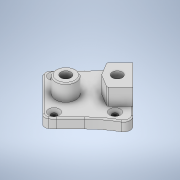
# Autodesk Inventor part: LegPin_Middle_v1
Saved by Autodesk Inventor 2020.3 (Build 243373000, 373)
## iProperties
Created: 2021-03-02
Part Number: LegPin_Middle_v1
Material: Generic
Document SubType Name: Modeling
Designer: sanyi
Density: 1 g/cm^3
Appearance: Default
Author: sanyi
Autodesk Inventor part; units mm, degrees
ref_plane "YZ Plane" through (0, 0, 0) normal (1, 0, 0) x (0, 1, 0)
ref_plane "XZ Plane" through (0, 0, 0) normal (0, 1, 0) x (-1, 0, 0)
ref_plane "XY Plane" through (0, 0, 0) normal (0, 0, 1) x (1, 0, 0)
sketch "Sketch1" plane through (0, 0, 0) normal (0, 1, 0) x (-1, 0, 0)
  line L0 (0, 114.5515) -> (0, -115.3375) construction
  line L1 (119.911, 0) -> (-136.2846, 0) construction
  line L2 (65, 45) -> (30.4932, 45) construction
  line L3 (-65, 45) -> (-65, 10.4932) construction
  line L4 (-65, -45) -> (-19.7, -45) construction
  line L5 (65, -45) -> (65, -10.4932) construction
  line L6 (64.2599, -35.4918) -> (81.6548, -52.8866) construction
  line L7 (81.6548, -52.8866) -> (72.8866, -61.6548) construction
  line L8 (72.8866, -61.6548) -> (55.4918, -44.2599) construction
  line L9 (55.4918, -44.2599) -> (64.2599, -35.4918) construction
  line L10 (64.2599, 35.4918) -> (81.6548, 52.8866)
  line L11 (81.6548, 52.8866) -> (72.8866, 61.6548)
  line L12 (72.8866, 61.6548) -> (55.4918, 44.2599)
  line L13 (55.4918, 44.2599) -> (59.8759, 39.8759)
  line L14 (-55.4918, 44.2599) -> (-72.8866, 61.6548) construction
  line L15 (-72.8866, 61.6548) -> (-81.6548, 52.8866) construction
  line L16 (-81.6548, 52.8866) -> (-64.2599, 35.4918) construction
  line L17 (-64.2599, 35.4918) -> (-55.4918, 44.2599) construction
  line L18 (-55.4918, -44.2599) -> (-72.8866, -61.6548) construction
  line L19 (-72.8866, -61.6548) -> (-81.6548, -52.8866) construction
  line L20 (-81.6548, -52.8866) -> (-64.2599, -35.4918) construction
  line L21 (-64.2599, -35.4918) -> (-55.4918, -44.2599) construction
  line L22 (55, 30) -> (-15, 30) construction
  line L23 (-15, 30) -> (-15, -30) construction
  line L24 (-15, -30) -> (55, -30) construction
  line L25 (55, -30) -> (55, 30) construction
  line L26 (72.9574, 44.1892) -> (64.1892, 52.9574) construction
  line L27 (68.0783, 56.8464) -> (76.8464, 48.0783) construction
  circle A0 centre (72.4624, 52.4624) radius 4.25
  line L28 (72.9574, -44.1892) -> (64.1892, -52.9574) construction
  line L29 (76.8464, -48.0783) -> (68.0783, -56.8464) construction
  circle A1 centre (72.4624, -52.4624) radius 4.25 construction
  line L30 (-64.1892, 52.9574) -> (-72.9574, 44.1892) construction
  line L31 (-68.0783, 56.8464) -> (-76.8464, 48.0783) construction
  circle A2 centre (-72.4624, 52.4624) radius 4.25 construction
  line L32 (-72.9574, -44.1892) -> (-64.1892, -52.9574) construction
  line L33 (-76.8464, -48.0783) -> (-68.0783, -56.8464) construction
  circle A3 centre (-72.4624, -52.4624) radius 4.25 construction
  line L34 (6.8, 51.2) -> (-17.8, 51.2) construction
  line L35 (-17.8, 51.2) -> (-17.8, 38.8) construction
  line L36 (-17.8, 38.8) -> (6.8, 38.8) construction
  line L37 (6.8, 38.8) -> (6.8, 51.2) construction
  line L38 (6.8, -38.8) -> (-17.8, -38.8) construction
  line L39 (-17.8, -38.8) -> (-17.8, -51.2) construction
  line L40 (-17.8, -51.2) -> (6.8, -51.2) construction
  line L41 (6.8, -51.2) -> (6.8, -38.8) construction
  line L42 (6.8, 45) -> (-17.8, 45) construction
  line L43 (-5.5, 51.2) -> (-5.5, 38.8) construction
  line L44 (0, 51.2) -> (0, 38.8) construction
  line L45 (6.8, -45) -> (-17.8, -45) construction
  line L46 (-5.5, -38.8) -> (-5.5, -51.2) construction
  line L47 (0, -38.8) -> (0, -51.2) construction
  circle A4 centre (0, 45) radius 4.25 construction
  circle A5 centre (0, -45) radius 4.25 construction
  line L48 (20, 30) -> (20, -30) construction
  line L49 (8.8, 57.2) -> (-19.8, 57.2) construction
  line L50 (8.8, -57.2) -> (-19.8, -57.2) construction
  line L51 (8.8, 57.2) -> (8.8, 45) construction
  line L52 (-19.8, 57.2) -> (-19.8, 45) construction
  line L53 (8.8, -57.2) -> (8.8, -45) construction
  line L54 (-19.8, -57.2) -> (-19.8, -45) construction
  line L55 (65.8156, 63.069) -> (59.9466, 57.2)
  line L56 (83.069, 45.8156) -> (77.2, 39.9466)
  line L57 (64.1892, 52.9574) -> (59.9466, 57.2) construction
  line L58 (72.9574, 44.1892) -> (77.2, 39.9466) construction
  arc A6 (83.069, 45.8156) -> (65.8156, 63.069) centre (74.4423, 54.4423) ccw
  line L59 (-59.9466, 57.2) -> (-65.8156, 63.069) construction
  line L60 (-83.069, 45.8156) -> (-77.2, 39.9466) construction
  line L61 (-59.9466, 57.2) -> (-64.1892, 52.9574) construction
  line L62 (-77.2, 39.9466) -> (-72.9574, 44.1892) construction
  arc A7 (-65.8156, 63.069) -> (-83.069, 45.8156) centre (-74.4423, 54.4423) ccw construction
  line L63 (72.9574, -44.1892) -> (77.2, -39.9466) construction
  line L64 (77.2, -39.9466) -> (83.069, -45.8156) construction
  line L65 (64.1892, -52.9574) -> (59.9466, -57.2) construction
  line L66 (59.9466, -57.2) -> (65.8156, -63.069) construction
  arc A8 (65.8156, -63.069) -> (83.069, -45.8156) centre (74.4423, -54.4423) ccw construction
  line L67 (-72.9574, -44.1892) -> (-77.2, -39.9466) construction
  line L68 (-64.1892, -52.9574) -> (-59.9466, -57.2) construction
  line L69 (-59.9466, -57.2) -> (-65.8156, -63.069) construction
  line L70 (-77.2, -39.9466) -> (-83.069, -45.8156) construction
  arc A9 (-83.069, -45.8156) -> (-65.8156, -63.069) centre (-74.4423, -54.4423) ccw construction
  arc A10 (23.5363, -45) -> (8.8, -57.2) centre (23.5363, -60) ccw construction
  arc A11 (59.9466, -57.2) -> (30.4932, -45) centre (30.4932, -86.6534) ccw construction
  arc A12 (65, -10.4932) -> (77.2, -39.9466) centre (106.6534, -10.4932) ccw construction
  arc A13 (77.2, 39.9466) -> (65, 10.4932) centre (106.6534, 10.4932) ccw
  arc A14 (30.4932, 45) -> (59.9466, 57.2) centre (30.4932, 86.6534) ccw
  arc A15 (8.8, 57.2) -> (23.5363, 45) centre (23.5363, 60) ccw construction
  arc A16 (-65, 10.4932) -> (-77.2, 39.9466) centre (-106.6534, 10.4932) ccw construction
  arc A17 (-77.2, -39.9466) -> (-65, -10.4932) centre (-106.6534, -10.4932) ccw construction
  line L71 (72.4624, -52.4624) -> (-72.4624, -52.4624) construction
  line L72 (-72.4624, 52.4624) -> (72.4624, 52.4624) construction
  line L73 (-59.9466, 57.2) -> (-59.9466, 45) construction
  line L74 (-59.9466, -57.2) -> (-59.9466, -45) construction
  arc A18 (-19.8, -57.2) -> (-34.5363, -45) centre (-34.5363, -60) ccw construction
  arc A19 (-30.4932, -45) -> (-59.9466, -57.2) centre (-30.4932, -86.6534) ccw construction
  arc A20 (-34.5363, 45) -> (-33.0208, 45.0768) centre (-34.5363, 60) ccw construction
  arc A21 (-59.9466, 57.2) -> (-33.0208, 45.0768) centre (-30.4932, 86.6534) ccw construction
  line L75 (72.8866, 61.6548) -> (75.7151, 64.4832) construction
  line L76 (75.7151, 64.4832) -> (84.4832, 55.7151) construction
  line L77 (84.4832, 55.7151) -> (81.6548, 52.8866) construction
  line L78 (78.6142, 58.6142) -> (58.5324, 38.5324) construction
  line L79 (58.5324, -38.5324) -> (78.6142, -58.6142) construction
  line L80 (-78.6142, 58.6142) -> (-58.5324, 38.5324) construction
  line L81 (-78.6142, -58.6142) -> (-58.5324, -38.5324) construction
  line L82 (74.4423, 54.4423) -> (77.2707, 57.2707) construction
  line L83 (74.4423, -54.4423) -> (77.2707, -57.2707) construction
  line L84 (-74.4423, -54.4423) -> (-77.2707, -57.2707) construction
  line L85 (-74.4423, 54.4423) -> (-77.2707, 57.2707) construction
  line L86 (-19.7, 45) -> (-65, 45) construction
  line L87 (8.7, 45) -> (-19.7, 45) construction
  line L88 (8.7, -45) -> (23.5363, -45) construction
  line L89 (-19.7, -45) -> (8.7, -45) construction
  line L90 (81.6548, 52.8866) -> (85.4206, 49.1209)
  line L91 (72.8866, 61.6548) -> (69.1209, 65.4206)
  line L92 (79.4627, 55.0787) -> (74.6544, 50.2704) construction
  line L93 (70.2704, -54.6544) -> (75.0787, -59.4627) construction
  line L94 (0, -48.1) -> (6.8, -48.1) construction
  line L95 (-74.6544, -50.2704) -> (-79.4627, -55.0787) construction
  line L96 (-75.0787, 59.4627) -> (-70.2704, 54.6544) construction
  line L97 (0, 48.1) -> (6.8, 48.1) construction
  line L98 (81.6548, -52.8866) -> (85.4206, -49.1209) construction
  line L99 (72.8866, -61.6548) -> (69.1209, -65.4206) construction
  line L100 (-72.8866, -61.6548) -> (-69.1209, -65.4206) construction
  line L101 (-81.6548, -52.8866) -> (-85.4206, -49.1209) construction
  line L102 (-72.8866, 61.6548) -> (-69.1209, 65.4206) construction
  line L103 (-81.6548, 52.8866) -> (-85.4206, 49.1209) construction
  line L104 (30.4932, 45) -> (23.5363, 45) construction
  line L105 (23.5363, 45) -> (8.7, 45) construction
  arc A22 (-33.0208, 45.0768) -> (-30.4932, 45) centre (-30.4932, 86.6534) ccw construction
  arc A23 (-33.0208, 45.0768) -> (-19.8, 57.2) centre (-34.5363, 60) ccw construction
  line L106 (-21.6459, 42) -> (-51.6459, 42) construction
  line L107 (-51.6459, 42) -> (-51.6459, -42) construction
  line L108 (-51.6459, -42) -> (-21.6459, -42) construction
  line L109 (-21.6459, -42) -> (-21.6459, 42) construction
  line L110 (52, 27) -> (55, 27) construction
  line L111 (52, -27) -> (55, -27) construction
  line L112 (52, 27) -> (52, 30) construction
  line L113 (-12, 27) -> (-12, 30) construction
  line L114 (-12, 27) -> (-15, 27) construction
  line L115 (-15, -27) -> (-12, -27) construction
  line L116 (-12, -27) -> (-12, -30) construction
  line L117 (52, -27) -> (52, -30) construction
  line L118 (-19.1459, 10) -> (-20.6459, 10) construction
  line L119 (-20.6459, 10) -> (-20.6459, -10) construction
  line L120 (-20.6459, -10) -> (-19.1459, -10) construction
  line L121 (-19.1459, -10) -> (-19.1459, 10) construction
  line L122 (-19.1459, 0) -> (-20.6459, 0) construction
  line L123 (-36.6459, 42) -> (-36.6459, -42) construction
  line L124 (-52.6459, 10) -> (-54.1459, 10) construction
  line L125 (-54.1459, 10) -> (-54.1459, -10) construction
  line L126 (-54.1459, -10) -> (-52.6459, -10) construction
  line L127 (-52.6459, -10) -> (-52.6459, 10) construction
  line L128 (-52.6459, 0) -> (-54.1459, 0) construction
  line L129 (30.4932, -45) -> (65, -45) construction
  line L130 (23.5363, -45) -> (30.4932, -45) construction
  line L131 (65, -10.4932) -> (65, 10.4932) construction
  line L132 (65, 10.4932) -> (65, 45) construction
  arc A24 (68.1707, 26.4333) -> (64.2599, 35.4918) centre (54.8044, 26.0363) ccw
  arc A25 (55.4918, 44.2599) -> (46.4333, 48.1707) centre (46.0363, 34.8044) ccw
  arc A26 (64.2599, -35.4918) -> (68.1707, -26.4333) centre (54.8044, -26.0363) ccw construction
  arc A27 (46.4333, -48.1707) -> (55.4918, -44.2599) centre (46.0363, -34.8044) ccw construction
  arc A28 (-55.4918, -44.2599) -> (-46.4333, -48.1707) centre (-46.0363, -34.8044) ccw construction
  arc A29 (-68.1707, -26.4333) -> (-64.2599, -35.4918) centre (-54.8044, -26.0363) ccw construction
  arc A30 (-47.594, 48.6723) -> (-55.4918, 44.2599) centre (-43.7511, 32.5192) ccw construction
  arc A31 (-64.2599, 35.4918) -> (-68.1707, 26.4333) centre (-54.8044, 26.0363) ccw construction
  line L133 (-65, 10.4932) -> (-65, -10.4932) construction
  line L134 (-65, -10.4932) -> (-65, -45) construction
  line L135 (-55.4918, 44.2599) -> (-55.4918, -44.2599) construction
  arc A32 (-19.9504, 56.5) -> (-17.8, 51.2) centre (-15.1706, 55.3531) ccw construction
  arc A33 (6.8, 51.2) -> (8.9504, 56.5) centre (4.1706, 55.3531) ccw construction
  arc A34 (8.9504, -56.5) -> (6.8, -51.2) centre (4.1706, -55.3531) ccw construction
  arc A35 (-17.8, -51.2) -> (-19.9504, -56.5) centre (-15.1706, -55.3531) ccw construction
  line L136 (-17.8, 38.8) -> (-17.8, 32.8) construction
  line L137 (-17.8, 32.8) -> (6.8, 32.8) construction
  line L138 (6.8, 32.8) -> (6.8, 38.8) construction
  line L139 (-17.8, -38.8) -> (-17.8, -32.8) construction
  line L140 (-17.8, -32.8) -> (6.8, -32.8) construction
  line L141 (6.8, -32.8) -> (6.8, -38.8) construction
  line L142 (81.4426, 48.4319) -> (68.4319, 61.4426) construction
  line L143 (68.4319, 61.4426) -> (55.704, 48.7147) construction
  line L144 (55.704, 48.7147) -> (68.7147, 35.704) construction
  line L145 (68.7147, 35.704) -> (81.4426, 48.4319) construction
  line L146 (65, 45) -> (59.5223, 48.2905)
  line L147 (65, 45) -> (68.2905, 39.5223)
  line L148 (68.2905, 39.5223) -> (59.5223, 48.2905) construction
  circle A36 centre (72.4624, 52.4624) radius 3.6
  line L149 (63.2232, 40.2385) -> (60.077, 43.3846)
  line L150 (59.8759, 39.8759) -> (64.2599, 35.4918)
  circle A37 centre (61.7308, 41.7308) radius 2.8
  arc A38 (51.3061, 50.5725) -> (51.4898, 47.014) centre (52.3054, 48.8401) ccw construction
  arc A39 (67.014, 31.4898) -> (70.5725, 31.3061) centre (68.8401, 32.3054) ccw construction
  line L151 (50.7289, 46.1945) -> (66.1945, 30.7289)
  arc A40 (66.1945, 30.7289) -> (70.5725, 31.3061) centre (68.1621, 32.6965) ccw
  arc A41 (51.3061, 50.5725) -> (50.7289, 46.1945) centre (52.6965, 48.1621) ccw
  line L152 (55.4918, 44.2599) -> (54.0776, 42.8457)
  line L153 (64.2599, 35.4918) -> (62.8457, 34.0776)
  line L154 (58.5324, 38.5324) -> (58.4617, 38.4617) construction
  point P0 (0, 0)
  point P1 (65.0004, 0)
  point P2 (55, 0)
  point P3 (59.8759, -39.8759)
  point P4 (-59.8759, 39.8759)
  point P5 (-58.5324, -38.5324)
  point P6 (-59.8759, -39.8759)
  point P7 (0, 45)
  point P8 (-33.9298, 45.0048)
  point P9 (-33.0208, -45.0768)
  point P10 (-54.6887, -45)
  point P11 (-56.2319, -45)
  point P12 (-56.2319, 45)
  point P13 (-54.7019, 45)
  dimension "d0" = 135
  dimension "d4" = 24.6
  dimension "d5" = 12.4
  dimension "d6" = 70
  dimension "d7" = 60
  dimension "d9" = 8.5
  dimension "d10" = 135
  dimension "d12" = 6
  dimension "d13" = 2
  dimension "d14" = 2
  dimension "d16" = 20
  dimension "d23" = 6
  dimension "d29" = 130
  dimension "d32" = 15
  dimension "d33" = 4
  dimension "d34" = 28.4
  dimension "d38" = 4
  dimension "d40" = 6.8
  dimension "d49" = 30
  dimension "d50" = 84
  dimension "d51" = 3
  dimension "d52" = 3
  dimension "d53" = 1.5
  dimension "d54" = 20
  dimension "d59" = 1
  dimension "d60" = 90
  dimension "d61" = 135
  dimension "d70" = 135
  dimension "d82" = 0.7
  dimension "d83" = 0.7
  dimension "d84" = 0.7
  dimension "d85" = 0.7
  dimension "d86" = 6
  dimension "d108" = 18
  dimension "d134" = 5.7
  dimension "d135" = 7.2
  dimension "d143" = 5.6
  dimension "d166" = 2
  dimension "d167" = 2
  constraints: 308 end point, 97 tangent, 92 point on circle, 84 point on line, 83 perpendicular, 70 parallel, 43 midpoint, 42 centre point, 40 equal length, 18 horizontal, 15 collinear, 12 coincident, 9 equal radius, 8 symmetric about line, 3 vertical, 33 other
  measures "d0" angle of L3 L16
  measures "d4" distance between parallel lines of L11 L13
  measures "d5" distance between parallel lines of L10 L12
  measures "d6" distance of L24.end L23.end
  measures "d7" distance of L23.end L22.end
  measures "d9" diameter of A0
  measures "d10" angle of L6 L5
  measures "d12" distance between parallel lines of L34 L49
  measures "d13" distance between parallel lines of L37 L51
  measures "d14" distance between parallel lines of L41 L53
  measures "d16" distance between parallel lines of L0 L48
  measures "d23" distance between parallel lines of L56 L10
  measures "d29" distance between parallel lines of L3 L5
  measures "d32" radius of A15
  measures "d33" distance between parallel lines of L76 L11
  measures "d34" distance of L78.start L78.end
  measures "d38" distance of L82.start L82.end
  measures "d40" distance between parallel lines of L11 L27
  measures "d49" distance of L108.end L107.end
  measures "d50" distance of L107.end L106.end
  measures "d51" distance of L110.start L110.end
  measures "d52" distance of L110.start L112.end
  measures "d53" distance of L120.end L119.end
  measures "d54" distance of L119.end L118.end
  measures "d59" distance between parallel lines of L109 L119
  measures "d60" distance between parallel lines of L2 L88
  measures "d61" angle of L132 L10
  measures "d70" angle of L134 L20
  measures "d82" vertical distance of L49.end A32.start
  measures "d83" vertical distance of L49.start A33.end
  measures "d84" vertical distance of L50.start A34.start
  measures "d85" vertical distance of L50.end A35.end
  measures "d86" distance between parallel lines of L36 L137
  measures "d108" distance of L144.end L142.start
  measures "d134" distance between parallel lines of L148 L13
  measures "d135" diameter of A36
  measures "d143" diameter of A37
  measures "d166" radius of A38
  measures "d167" distance between parallel lines of L151 L13
extrude "Extrusion12" add sketch "Sketch1" along normal blind 4 contours L10 L90 A6 L56 A13 A40 A24 | A24 A40 L151 L153 | L151 A41 A25 L152 | L12 A25 A41 A14 L55 A6 L91
extrude "Extrusion13" add sketch "Sketch1" along normal blind 4 contours L147 L146 L12 L11 L10
extrude "Extrusion14" add sketch "Sketch1" along normal blind 10.9 contours A0 | A36
extrude "Extrusion15" add sketch "Sketch1" along normal blind 10.9 contours L150 A37 L13 L12 L146 L147 L10 | L153 L151 L152 L13 A37 L150 | A37 L13 L150 | L150 L13 A37
sketch "Sketch3" plane through (0, 10.9, 0) normal (0, 1, 0) x (1, 0, 0)
  line L0 (-68.2905, -39.5223) -> (-65, -45) projected
  line L1 (-65, -45) -> (-59.5223, -48.2905) projected
  line L2 (-68.2905, -39.5223) -> (-65, -45) projected
  line L3 (-65, -45) -> (-58.4617, -38.4617) construction
  line L4 (-64.9493, -38.5124) -> (-58.4843, -44.9774) construction
  line L5 (-62.8457, -34.0776) -> (-68.2905, -39.5223) projected
  line L6 (-59.5223, -48.2905) -> (-54.0776, -42.8457) projected
  line L7 (-54.0776, -42.8457) -> (-62.8457, -34.0776) projected
  point P0 (0, 0)
  point P1 (-61.7308, -41.7308)
  constraints: 4 end point, 2 midpoint, 1 point on line, 1 symmetric about line
fillet "Fillet10" radius 2 2 edges at (-85.4206, 2, 49.1209) (-69.1209, 2, 65.4206)
fillet "Fillet11" radius 0.5 12 edges at (-55.8439, 4, 53.6027) (-62.8811, 4, 60.1345) (-66.7074, 4, 63.8769) (-68.9811, 4, 64.9192) (-73.6027, 4, 35.8439) (-80.1345, 4, 42.8811) (-83.8769, 4, 46.7074) (-84.9192, 4, 48.9811) (-68.2124, 10.9, 52.4624) (-59.5223, 7.45, 48.2905) (-65, 7.45, 45) (-68.2905, 7.45, 39.5223)
sketch "Sketch2" plane through (-72.4624, 10.9, 52.4624) normal (0, 1, 0) x (1, 0, 0)
  circle A0 centre (0, 0) radius 4.25 projected
  point P0 (72.4624, 52.4624)
  constraints: 1 coincident
hole "Hole3" at (-72.4624, 10.9, 52.4624) direction (0, -1, 0) diameter 4.2 depth 10.9
hole "Hole5" at (-61.7308, 10.9, 41.7308) direction (0, -1, 0) diameter 4.2 depth 10.9
hole "Hole6" at (-72.4624, 0, -52.4624) at (72.4624, 0, 52.4624) at (72.4624, 0, -52.4624) at (0, 0, 45) at (0, 0, -45) at (78.6142, 0, 58.6142) at (78.6142, 0, -58.6142) at (-58.5324, 0, -38.5324) at (-78.6142, 0, -58.6142) at (58.5324, 0, 38.5324) at (58.5324, 0, -38.5324) at (-8.7, 0, 45) at (19.7, 0, 45) at (-8.7, 0, -45) at (19.7, 0, -45) at (12, 0, 27) at (12, 0, -27) at (-52, 0, -27) at (-52, 0, 27) at (-72.4624, 0, 52.4624) at (-61.7308, 0, 41.7308) direction (0, 1, 0) diameter 5.6 depth 6.5 counterbore diameter 9 counterbore depth 1
sketch "Sketch5" plane through (0, 4, 0) normal (0, 1, 0) x (1, 0, 0)
  point P0 (0, 0)
  point P1 (-68.4319, -61.4426)
  point P2 (-55.704, -48.7147)
  point P3 (-68.7147, -35.704)
  point P4 (-81.4426, -48.4319)
hole "Hole7" at (-68.4319, 4, 61.4426) at (-55.704, 4, 48.7147) at (-68.7147, 4, 35.704) at (-81.4426, 4, 48.4319) direction (0, -1, 0) diameter 2.3 depth 6.5 countersink diameter 4.5 countersink angle 90
body "Solid6"
